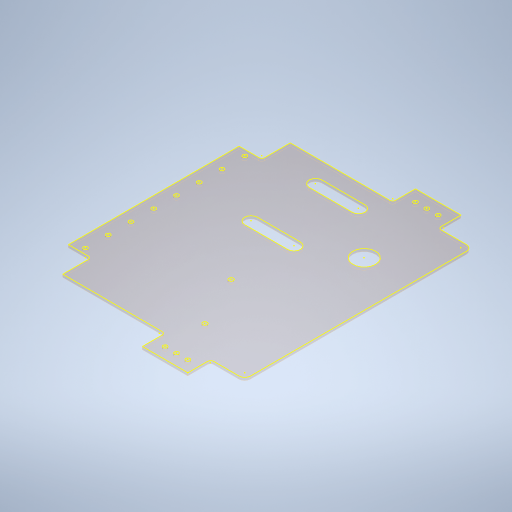
# Autodesk Inventor part: 1561 Daughter Board
Saved by Autodesk Inventor 2023.3 (Build 273359000, 359)
## iProperties
Created: 2023-10-01
Part Number: 1561 Daughter Board
Material: Generic
Document SubType Name: Modeling
Designer: jackc
Density: 1 g/cm^3
Appearance: Polycarbonate - Smoked
Author: jackc
Autodesk Inventor part; units mm, degrees
ref_plane "YZ Plane" through (0, 0, 0) normal (1, 0, 0) x (0, 1, 0)
ref_plane "XZ Plane" through (0, 0, 0) normal (0, 1, 0) x (-1, 0, 0)
ref_plane "XY Plane" through (0, 0, 0) normal (0, 0, 1) x (1, 0, 0)
sketch "Sketch1" plane through (0, 0, 0) normal (0, 1, 0) x (-1, 0, 0)
  line L0 (-38.1, -25.4) -> (-38.1, -279.4)
  line L1 (0, -304.8) -> (50.8, -304.8)
  line L2 (50.8, -304.8) -> (50.8, -279.4)
  line L3 (50.8, -279.4) -> (190.5, -279.4)
  line L4 (190.5, -279.4) -> (190.5, -25.4)
  line L5 (190.5, -25.4) -> (50.8, -25.4)
  line L6 (50.8, -25.4) -> (50.8, 0)
  line L7 (50.8, 0) -> (0, 0)
  circle A0 centre (38.1, -12.7) radius 2.3622
  circle A1 centre (25.4, -12.7) radius 2.3622
  circle A2 centre (12.7, -12.7) radius 2.3622
  line L8 (-38.1, -152.4) -> (190.5, -152.4) construction
  circle A3 centre (177.8, -139.7) radius 2.3622
  circle A4 centre (177.8, -114.3) radius 2.3622
  circle A5 centre (177.8, -88.9) radius 2.3622
  circle A6 centre (177.8, -63.5) radius 2.3622
  circle A7 centre (38.1, -292.1) radius 2.3622
  circle A8 centre (25.4, -292.1) radius 2.3622
  circle A9 centre (12.7, -292.1) radius 2.3622
  circle A10 centre (177.8, -165.1) radius 2.3622
  circle A11 centre (177.8, -190.5) radius 2.3622
  circle A12 centre (177.8, -215.9) radius 2.3622
  circle A13 centre (177.8, -241.3) radius 2.3622
  line L9 (0, 0) -> (0, -25.4)
  line L10 (0, -25.4) -> (-38.1, -25.4)
  line L11 (-38.1, -279.4) -> (0, -279.4)
  line L12 (0, -279.4) -> (0, -304.8)
  line L13 (190.5, -57.15) -> (165.1, -57.15)
  line L14 (165.1, -57.15) -> (165.1, -25.4)
  line L15 (190.5, -247.65) -> (165.1, -247.65)
  line L16 (165.1, -247.65) -> (165.1, -279.4)
  circle A14 centre (66.04, -114.3) radius 2.5527
  circle A15 centre (38.1, -57.15) radius 2.5527
  circle A16 centre (12.7, -209.55) radius 12.7
  circle A17 centre (12.7, -209.55) radius 28.575 construction
  line L17 (111.5, -254) -> (111.5, -182) construction
  line L18 (111.5, -182) -> (63.5, -182) construction
  line L19 (63.5, -182) -> (63.5, -254) construction
  line L20 (63.5, -254) -> (111.5, -254) construction
  line L21 (111.5, -254) -> (63.5, -254) construction
  line L22 (111.5, -246.8562) -> (63.5, -246.8562)
  line L23 (63.5, -261.1437) -> (111.5, -261.1437)
  arc A18 (111.5, -261.1437) -> (111.5, -246.8562) centre (111.5, -254) ccw
  arc A19 (63.5, -246.8562) -> (63.5, -261.1437) centre (63.5, -254) ccw
  line L24 (111.5, -182) -> (63.5, -182) construction
  line L25 (111.5, -174.8562) -> (63.5, -174.8562)
  line L26 (63.5, -189.1437) -> (111.5, -189.1437)
  arc A20 (111.5, -189.1437) -> (111.5, -174.8562) centre (111.5, -182) ccw
  arc A21 (63.5, -174.8562) -> (63.5, -189.1437) centre (63.5, -182) ccw
  point P0 (177.8, -279.4)
  point P1 (120.65, -279.4)
  point P2 (87.5, -254)
  point P3 (87.5, -182)
  dimension "d0" = 254
  dimension "d1" = 50.8
  dimension "d2" = 25.4
  dimension "d4" = 12.7
  dimension "d5" = 12.7
  dimension "d6" = 12.7
  dimension "d7" = 12.7
  dimension "d8" = 4.7244
  dimension "d9" = 12.7
  dimension "d10" = 12.7
  dimension "d13" = 25.4
  dimension "d20" = 228.6
  dimension "d21" = 38.1
  dimension "d22" = 25.4
  dimension "d23" = 6.35
  dimension "d25" = 5.1054
  dimension "d28" = 57.15
  dimension "d29" = 27.94
  dimension "d31" = 25.4
  dimension "d32" = 57.15
  dimension "d33" = 152.4
  dimension "d34" = 69.85
  dimension "d35" = 72
  dimension "d36" = 48
  dimension "d37" = 14.2875
  dimension "d38" = 14.2875
  dimension "d42" = 38.1
  dimension "d43" = 31.75
  dimension "d44" = 0
  dimension "d45" = 25.4
  dimension "d46" = 63.5
  constraints: 58 end point, 22 centre point, 11 perpendicular, 8 point on circle, 8 tangent, 7 point on line, 7 symmetric about line, 5 midpoint, 5 parallel, 4 equal radius, 4 horizontal alignment, 4 vertical, 3 equal length, 2 horizontal, 1 coincident, 1 collinear, 1 vertical alignment, 13 other
  measures "d0" distance of L0.end L0.start
  measures "d1" distance of L1.start L1.end
  measures "d2" distance of L1.end L2.end
  measures "d4" distance from line of A1.centre L7
  measures "d5" distance of A0.centre A1.centre
  measures "d6" distance of A1.centre A2.centre
  measures "d7" distance from line of L6 A0.centre
  measures "d8" diameter of A1
  measures "d9" distance from line of L4 A3.centre
  measures "d10" distance from line of A3.centre L8
  measures "d13" distance of A3.centre A4.centre
  measures "d20" distance between parallel lines of L4 L0
  measures "d21" distance of L9.end L0.start
  measures "d22" distance between parallel lines of L14 L4
  measures "d23" distance from line of A13.centre L15
  measures "d25" diameter of A14
  measures "d28" vertical distance of A15.centre A14.centre
  measures "d29" horizontal distance of A14.centre A15.centre
  measures "d31" diameter of A16
  measures "d32" diameter of A17
  measures "d33" distance from line of L16 A16.centre
  measures "d34" vertical distance of point (120.65, -279.4) A16.centre
  measures "d35" distance of L17.start L17.end
  measures "d36" distance of L19.end L17.start
  measures "d37" distance between parallel lines of L23 L22
  measures "d38" diameter of A21
  measures "d42" horizontal distance of A15.centre L9.end
  measures "d43" distance from line of L5 A15.centre
  measures "d44" angle of L3 L20
  measures "d45" distance from line of point (120.65, -279.4) L20
  measures "d46" horizontal distance of L11.end L19.end
extrude "Extrusion1" add sketch "Sketch1" along normal blind 3.175 contours L10 L9 L7 L6 L5 L14 L13 L4 L15 L16 L3 L2 L1 L12 L11 L0
fillet "Fillet1" radius 3.175 6 edges at (-165.1, 1.5875, -57.15) (-165.1, 1.5875, -247.65) (-50.8, 1.5875, -279.4) (0, 1.5875, -279.4) (0, 1.5875, -25.4) (-50.8, 1.5875, -25.4)
fillet "Fillet2" radius 6.35 2 edges at (38.1, 1.5875, -25.4) (38.1, 1.5875, -279.4)
sketch "Cut Sketch" plane through (0, 3.175, 0) normal (0, 1, 0) x (1, 0, 0)
  arc A0 (38.1, 273.05) -> (31.75, 279.4) centre (31.75, 273.05) ccw projected
  line L0 (31.75, 279.4) -> (3.175, 279.4) projected
  arc A1 (0, 282.575) -> (3.175, 279.4) centre (3.175, 282.575) ccw projected
  line L1 (0, 282.575) -> (0, 304.8) projected
  line L2 (0, 304.8) -> (-50.8, 304.8) projected
  line L3 (-50.8, 304.8) -> (-50.8, 282.575) projected
  arc A2 (-53.975, 279.4) -> (-50.8, 282.575) centre (-53.975, 282.575) ccw projected
  line L4 (-53.975, 279.4) -> (-165.1, 279.4) projected
  line L5 (-165.1, 279.4) -> (-165.1, 250.825) projected
  arc A3 (-168.275, 247.65) -> (-165.1, 250.825) centre (-168.275, 250.825) ccw projected
  line L6 (-168.275, 247.65) -> (-190.5, 247.65) projected
  line L7 (-190.5, 247.65) -> (-190.5, 57.15) projected
  line L8 (-190.5, 57.15) -> (-168.275, 57.15) projected
  arc A4 (-165.1, 53.975) -> (-168.275, 57.15) centre (-168.275, 53.975) ccw projected
  line L9 (-165.1, 53.975) -> (-165.1, 25.4) projected
  line L10 (-165.1, 25.4) -> (-53.975, 25.4) projected
  arc A5 (-50.8, 22.225) -> (-53.975, 25.4) centre (-53.975, 22.225) ccw projected
  line L11 (-50.8, 22.225) -> (-50.8, 0) projected
  line L12 (-50.8, 0) -> (0, 0) projected
  line L13 (0, 0) -> (0, 22.225) projected
  arc A6 (3.175, 25.4) -> (0, 22.225) centre (3.175, 22.225) ccw projected
  line L14 (3.175, 25.4) -> (31.75, 25.4) projected
  arc A7 (31.75, 25.4) -> (38.1, 31.75) centre (31.75, 31.75) ccw projected
  line L15 (38.1, 31.75) -> (38.1, 273.05) projected
  circle A8 centre (-12.7, 209.55) radius 12.7 projected
  circle A9 centre (-66.04, 114.3) radius 2.5527 projected
  circle A10 centre (-25.4, 292.1) radius 2.3622 projected
  circle A11 centre (-177.8, 165.1) radius 2.3622 projected
  circle A12 centre (-177.8, 215.9) radius 2.3622 projected
  circle A13 centre (-177.8, 63.5) radius 2.3622 projected
  circle A14 centre (-177.8, 88.9) radius 2.3622 projected
  circle A15 centre (-177.8, 114.3) radius 2.3622 projected
  circle A16 centre (-177.8, 139.7) radius 2.3622 projected
  circle A17 centre (-12.7, 12.7) radius 2.3622 projected
  circle A18 centre (-25.4, 12.7) radius 2.3622 projected
  circle A19 centre (-38.1, 12.7) radius 2.3622 projected
  circle A20 centre (-177.8, 241.3) radius 2.3622 projected
  circle A21 centre (-177.8, 190.5) radius 2.3622 projected
  circle A22 centre (-38.1, 292.1) radius 2.3622 projected
  circle A23 centre (-12.7, 292.1) radius 2.3622 projected
  circle A24 centre (-38.1, 57.15) radius 2.5527 projected
  arc A25 (-111.5, 189.1437) -> (-111.5, 174.8562) centre (-111.5, 182) ccw projected
  line L16 (-111.5, 189.1437) -> (-63.5, 189.1437) projected
  arc A26 (-63.5, 174.8562) -> (-63.5, 189.1437) centre (-63.5, 182) ccw projected
  line L17 (-63.5, 174.8562) -> (-111.5, 174.8562) projected
  arc A27 (-111.5, 261.1437) -> (-111.5, 246.8562) centre (-111.5, 254) ccw projected
  line L18 (-111.5, 261.1437) -> (-63.5, 261.1437) projected
  arc A28 (-63.5, 246.8562) -> (-63.5, 261.1437) centre (-63.5, 254) ccw projected
  line L19 (-63.5, 246.8562) -> (-111.5, 246.8562) projected
body "Solid1"
